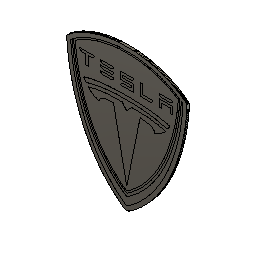
Tesla Shield Multipart (Autodesk Fusion 360 design; units mm, degrees)
Autodesk Fusion 360 part; units mm, degrees
(part 1 of 3)
sketch "Tesla Shield" plane through (0, 0, 0) normal (0, 0, 1) x (1, 0, 0)
  line L0 (187.3472, 241.9811) -> (187.8279, 240.6292)
  line L1 (217.7382, 211.8612) -> (216.8697, 213.1105)
  line L2 (210.0287, 224.007) -> (209.4066, 225.0419)
  line L3 (226.1937, 201.0406) -> (225.1992, 202.2018)
  line L4 (206.605, 201.6349) -> (207.38, 200.4172)
  line L5 (185.9594, 246.0449) -> (186.4129, 244.6891)
  line L6 (196.7783, 219.3402) -> (197.4176, 218.0403)
  line L7 (208.9597, 198.0038) -> (209.7645, 196.8085)
  line L8 (211.4038, 194.4412) -> (212.2385, 193.2697)
  line L9 (225.9747, 176.798) -> (226.9727, 175.7815)
  line L10 (228.9998, 173.7824) -> (230.029, 172.8002)
  line L11 (201.773, 240.4243) -> (201.2849, 241.5783)
  line L12 (192.5686, 228.5557) -> (193.1417, 227.228)
  line L13 (185.0795, 248.7587) -> (185.5149, 247.4014)
  line L14 (194.3162, 224.5831) -> (194.9175, 223.2662)
  line L15 (200.8071, 242.7368) -> (199.8754, 245.0637)
  line L16 (209.4066, 225.0419) -> (208.7947, 226.0826)
  line L17 (184.653, 250.1165) -> (185.0795, 248.7587)
  line L18 (224.218, 203.374) -> (223.2505, 204.5568)
  line L19 (193.7243, 225.9038) -> (194.3162, 224.5831)
  line L20 (197.4176, 218.0403) -> (198.0664, 216.745)
  line L21 (220.2044, 183.1227) -> (221.1404, 182.0426)
  line L22 (189.3251, 236.5837) -> (189.8425, 235.2392)
  line L23 (221.1404, 182.0426) -> (222.0866, 180.9727)
  line L24 (218.3631, 185.3125) -> (219.2786, 184.2127)
  line L25 (213.0832, 192.1065) -> (213.9379, 190.9519)
  line L26 (208.7947, 226.0826) -> (208.4968, 226.6074)
  line L27 (185.5149, 247.4014) -> (185.9594, 246.0449)
  line L28 (192.0048, 229.8867) -> (192.5686, 228.5557)
  line L29 (200.7575, 211.6148) -> (201.4543, 210.3458)
  line L30 (201.4543, 210.3458) -> (202.1609, 209.0826)
  line L31 (212.4736, 219.9224) -> (211.5554, 221.4433)
  line L32 (202.7875, 238.1331) -> (202.2733, 239.2756)
  line L33 (246.8929, 159.2455) -> (247.0305, 159.1815)
  line L34 (191.4503, 231.2207) -> (192.0048, 229.8867)
  line L35 (202.8772, 207.8253) -> (203.6032, 206.5742)
  line L36 (236.2567, 167.2973) -> (237.1439, 166.5675)
  line L37 (188.3178, 239.2788) -> (188.8169, 237.9302)
  line L38 (213.4053, 218.4097) -> (212.4736, 219.9224)
  line L39 (227.981, 174.7763) -> (228.9998, 173.7824)
  line L40 (205.0845, 204.0912) -> (205.8398, 202.8596)
  line L41 (195.5283, 221.9533) -> (196.1486, 220.6446)
  line L42 (220.4307, 208.1662) -> (219.5188, 209.3888)
  line L43 (186.4129, 244.6891) -> (186.8755, 243.3345)
  line L44 (189.8425, 235.2392) -> (190.3692, 233.8971)
  line L45 (188.8169, 237.9302) -> (189.3251, 236.5837)
  line L46 (202.2733, 239.2756) -> (201.773, 240.4243)
  line L47 (186.8755, 243.3345) -> (187.3472, 241.9811)
  line L48 (194.9175, 223.2662) -> (195.5283, 221.9533)
  line L49 (193.1417, 227.228) -> (193.7243, 225.9038)
  line L50 (227.2015, 199.8907) -> (226.1937, 201.0406)
  line L51 (198.7247, 215.4547) -> (199.3927, 214.1694)
  line L52 (190.9051, 232.5575) -> (191.4503, 231.2207)
  line L53 (216.8697, 213.1105) -> (216.0159, 214.3681)
  line L54 (214.3531, 216.9072) -> (213.4053, 218.4097)
  line L55 (208.4968, 226.6074) -> (208.2063, 227.1364)
  line L56 (199.8754, 245.0637) -> (198.9639, 247.3984)
  line L57 (211.5554, 221.4433) -> (210.648, 222.9706)
  line L58 (223.2505, 204.5568) -> (222.2966, 205.7499)
  line L59 (201.2849, 241.5783) -> (200.8071, 242.7368)
  line L60 (200.0703, 212.8894) -> (200.7575, 211.6148)
  line L61 (245.9016, 159.8961) -> (246.3605, 159.5744)
  line L62 (225.1992, 202.2018) -> (224.218, 203.374)
  line L63 (216.0159, 214.3681) -> (215.177, 215.6338)
  line L64 (213.9379, 190.9519) -> (214.8027, 189.8059)
  line L65 (245.3558, 160.2891) -> (245.9016, 159.8961)
  line L66 (246.7357, 159.3331) -> (246.8929, 159.2455)
  line L67 (234.5005, 168.7781) -> (235.3754, 168.0341)
  line L68 (216.5626, 187.5407) -> (217.4578, 186.4219)
  line L69 (207.38, 200.4172) -> (208.1649, 199.2068)
  line L70 (224.01, 178.864) -> (224.9872, 177.8256)
  line L71 (235.3754, 168.0341) -> (236.2567, 167.2973)
  line L72 (240.7476, 163.7156) -> (241.6609, 163.0186)
  line L73 (233.6321, 169.5295) -> (234.5005, 168.7781)
  line L74 (203.6032, 206.5742) -> (204.3389, 205.3294)
  line L75 (239.8389, 164.4189) -> (240.7476, 163.7156)
  line L76 (241.6609, 163.0186) -> (243.5005, 161.6424)
  line L77 (205.8398, 202.8596) -> (206.605, 201.6349)
  line L78 (226.9727, 175.7815) -> (227.981, 174.7763)
  line L79 (243.5005, 161.6424) -> (245.3558, 160.2891)
  line L80 (209.7645, 196.8085) -> (210.5791, 195.6209)
  line L81 (237.1439, 166.5675) -> (238.0368, 165.8447)
  line L82 (238.9353, 165.1285) -> (239.8389, 164.4189)
  line L83 (210.5791, 195.6209) -> (211.4038, 194.4412)
  line L84 (215.6776, 188.6688) -> (216.5626, 187.5407)
  line L85 (231.9159, 171.0551) -> (232.7705, 170.2885)
  line L86 (223.0431, 179.9131) -> (224.01, 178.864)
  line L87 (217.4578, 186.4219) -> (218.3631, 185.3125)
  line L88 (222.0866, 180.9727) -> (223.0431, 179.9131)
  line L89 (231.0687, 171.8297) -> (231.9159, 171.0551)
  line L90 (246.3605, 159.5744) -> (246.7357, 159.3331)
  line L91 (219.2786, 184.2127) -> (220.2044, 183.1227)
  line L92 (208.1649, 199.2068) -> (208.9597, 198.0038)
  line L93 (238.0368, 165.8447) -> (238.9353, 165.1285)
  line L94 (230.029, 172.8002) -> (231.0687, 171.8297)
  line L95 (212.2385, 193.2697) -> (213.0832, 192.1065)
  line L96 (214.8027, 189.8059) -> (215.6776, 188.6688)
  line L97 (232.7705, 170.2885) -> (233.6321, 169.5295)
  line L98 (224.9872, 177.8256) -> (225.9747, 176.798)
  line L99 (204.3389, 205.3294) -> (205.0845, 204.0912)
  line L100 (297.8145, 269.3775) -> (297.8286, 269.41)
  line L101 (206.9505, 271.3462) -> (206.1166, 271.1382)
  line L102 (220.5752, 273.5951) -> (218.9108, 273.3996)
  line L103 (244.7346, 273.0159) -> (244.2152, 273.6532)
  line L104 (200.9819, 269.6639) -> (200.9198, 269.6275)
  line L105 (293.8572, 265.8465) -> (294.3752, 266.2321)
  line L106 (263.8971, 274.4151) -> (262.0411, 274.448)
  line L107 (255.4396, 274.4952) -> (255.1595, 274.4828)
  line L108 (227.5104, 274.2394) -> (226.7191, 274.1886)
  line L109 (260.1865, 274.4663) -> (258.0237, 274.484)
  line L110 (201.2563, 268.8271) -> (201.3792, 268.686)
  line L111 (202.4895, 270.1206) -> (201.6512, 269.8782)
  line L112 (248.9154, 267.9355) -> (248.592, 268.3323)
  line L113 (226.7191, 274.1886) -> (225.7816, 274.1169)
  line L114 (243.5571, 274.4237) -> (243.4699, 274.5089)
  line L115 (249.1841, 267.626) -> (249.1226, 267.6892)
  line L116 (282.4148, 273.0309) -> (280.5744, 273.2723)
  line L117 (293.3298, 265.4726) -> (293.8572, 265.8465)
  line L118 (212.9583, 261.2685) -> (214.347, 260.9395)
  line L119 (265.7539, 274.3663) -> (263.8971, 274.4151)
  line L120 (219.1338, 266.4225) -> (219.4722, 266.55)
  line L121 (288.8178, 271.9664) -> (287.9073, 272.1405)
  line L122 (203.8665, 266.4028) -> (204.2509, 266.108)
  line L123 (212.8487, 272.5505) -> (212.0009, 272.4036)
  line L124 (297.8286, 269.41) -> (295.7733, 270.2687)
  line L125 (216.9125, 265.358) -> (217.2645, 265.5571)
  line L126 (202.0493, 267.9939) -> (202.3973, 267.6598)
  line L127 (208.7098, 263.3768) -> (209.7655, 262.8217)
  line L128 (269.4679, 274.2167) -> (267.611, 274.3005)
  line L129 (216.6366, 265.1892) -> (216.9125, 265.358)
  line L130 (249.1226, 267.6892) -> (248.9154, 267.9355)
  line L131 (200.9245, 269.36) -> (200.978, 269.2386)
  line L132 (295.8664, 267.4615) -> (296.3401, 267.8965)
  line L133 (267.611, 274.3005) -> (265.7539, 274.3663)
  line L134 (214.347, 260.9395) -> (214.6904, 262.7698)
  line L135 (216.2433, 264.9136) -> (216.4345, 265.0556)
  line L136 (289.7268, 271.7846) -> (288.8178, 271.9664)
  line L137 (203.1174, 267.0156) -> (203.4885, 266.7053)
  line L138 (258.0237, 274.484) -> (256.4399, 274.4982)
  line L139 (286.9953, 272.307) -> (286.0818, 272.4661)
  line L140 (294.3752, 266.2321) -> (294.8833, 266.6296)
  line L141 (297.5669, 269.108) -> (297.7654, 269.3164)
  line L142 (203.6318, 270.4539) -> (202.4895, 270.1206)
  line L143 (217.2645, 265.5571) -> (217.6947, 265.7815)
  line L144 (243.8236, 274.1236) -> (243.5571, 274.4237)
  line L145 (249.2182, 267.6047) -> (249.1841, 267.626)
  line L146 (248.1479, 268.8686) -> (247.0886, 270.1383)
  line L147 (295.3806, 267.0393) -> (295.8664, 267.4615)
  line L148 (200.8951, 269.4677) -> (200.9245, 269.36)
  line L149 (218.7986, 266.2867) -> (219.1338, 266.4225)
  line L150 (204.457, 270.6923) -> (203.6318, 270.4539)
  line L151 (255.0748, 274.4732) -> (255.0271, 274.461)
  line L152 (280.5744, 273.2723) -> (278.7301, 273.4878)
  line L153 (248.592, 268.3323) -> (248.1479, 268.8686)
  line L154 (209.4669, 271.9142) -> (208.6259, 271.734)
  line L155 (273.1788, 273.9905) -> (271.324, 274.1137)
  line L156 (201.7098, 268.3359) -> (202.0493, 267.9939)
  line L157 (287.9073, 272.1405) -> (286.9953, 272.307)
  line L158 (202.7535, 267.3338) -> (203.1174, 267.0156)
  line L159 (286.0818, 272.4661) -> (284.2508, 272.7625)
  line L160 (255.0271, 274.461) -> (249.2182, 267.6047)
  line L161 (262.0411, 274.448) -> (260.1865, 274.4663)
  line L162 (207.5087, 264.0243) -> (208.7098, 263.3768)
  line L163 (278.7301, 273.4878) -> (276.8823, 273.6786)
  line L164 (252.6831, 166.1124) -> (253.7398, 166.8931)
  line L165 (203.4885, 266.7053) -> (203.8665, 266.4028)
  line L166 (226.8539, 268.0985) -> (232.4298, 268.1876)
  line L167 (211.4348, 261.9774) -> (212.5034, 261.4676)
  line L168 (219.8135, 266.6699) -> (220.1574, 266.7825)
  line L169 (200.9023, 269.5956) -> (200.8926, 269.558)
  line L170 (218.2053, 266.0263) -> (218.7986, 266.2867)
  line L171 (212.5034, 261.4676) -> (212.9583, 261.2685)
  line L172 (232.5255, 268.105) -> (232.5909, 267.9917)
  line L173 (200.8926, 269.558) -> (200.8951, 269.4677)
  line L174 (250.0262, 164.2337) -> (250.3806, 164.4663)
  line L175 (204.2509, 266.108) -> (204.6414, 265.821)
  line L176 (273.2336, 184.725) -> (274.0907, 185.682)
  line L177 (232.4822, 268.1528) -> (232.5255, 268.105)
  line L178 (200.9198, 269.6275) -> (200.9023, 269.5956)
  line L179 (201.3792, 268.686) -> (201.7098, 268.3359)
  line L180 (206.1166, 271.1382) -> (205.2853, 270.9203)
  line L181 (201.6512, 269.8782) -> (201.1251, 269.717)
  line L182 (217.1017, 273.1756) -> (215.3984, 272.9463)
  line L183 (207.0877, 264.2585) -> (207.5087, 264.0243)
  line L184 (255.8253, 168.4921) -> (256.8568, 169.3066)
  line L185 (224.4041, 267.7293) -> (225.0148, 267.8346)
  line L186 (225.0148, 267.8346) -> (225.6259, 267.9391)
  line L187 (250.3806, 164.4663) -> (250.7648, 164.7364)
  line L188 (251.6155, 165.3469) -> (252.6831, 166.1124)
  line L189 (253.7398, 166.8931) -> (254.7867, 167.687)
  line L190 (215.3984, 272.9463) -> (213.6976, 272.6897)
  line L191 (200.978, 269.2386) -> (201.053, 269.1069)
  line L192 (205.0375, 265.5417) -> (205.4388, 265.27)
  line L193 (201.1251, 269.717) -> (200.9819, 269.6639)
  line L194 (202.3973, 267.6598) -> (202.7535, 267.3338)
  line L195 (210.3099, 272.0857) -> (209.4669, 271.9142)
  line L196 (205.4388, 265.27) -> (205.8449, 265.0059)
  line L197 (232.6262, 267.8904) -> (232.673, 267.7116)
  line L198 (249.1594, 163.8662) -> (249.2821, 163.8853)
  line L199 (249.5544, 163.9782) -> (249.7034, 164.0492)
  line L200 (221.5548, 267.1691) -> (222.2632, 267.3304)
  line L201 (219.4722, 266.55) -> (219.8135, 266.6699)
  line L202 (254.7867, 167.687) -> (255.8253, 168.4921)
  line L203 (225.6259, 267.9391) -> (226.2385, 268.0311)
  line L204 (250.7648, 164.7364) -> (251.6155, 165.3469)
  line L205 (218.9108, 273.3996) -> (217.1017, 273.1756)
  line L206 (214.6904, 262.7698) -> (216.2433, 264.9136)
  line L207 (212.0009, 272.4036) -> (211.1546, 272.2488)
  line L208 (213.6976, 272.6897) -> (212.8487, 272.5505)
  line L209 (206.2553, 264.7493) -> (206.6697, 264.5002)
  line L210 (210.6744, 262.3563) -> (211.4348, 261.9774)
  line L211 (247.7838, 192.4016) -> (248.8733, 187.0975)
  line L212 (216.4345, 265.0556) -> (216.6366, 265.1892)
  line L213 (272.4031, 183.8146) -> (273.2336, 184.725)
  line L214 (205.8449, 265.0059) -> (206.2553, 264.7493)
  line L215 (206.6697, 264.5002) -> (207.0877, 264.2585)
  line L216 (249.2821, 163.8853) -> (249.4139, 163.9231)
  line L217 (209.7655, 262.8217) -> (210.6744, 262.3563)
  line L218 (217.6947, 265.7815) -> (218.2053, 266.0263)
  line L219 (211.1546, 272.2488) -> (210.3099, 272.0857)
  line L220 (208.6259, 271.734) -> (207.787, 271.5448)
  line L221 (207.787, 271.5448) -> (206.9505, 271.3462)
  line L222 (201.1467, 268.9685) -> (201.2563, 268.8271)
  line L223 (204.6414, 265.821) -> (205.0375, 265.5417)
  line L224 (233.2192, 265.0188) -> (233.8646, 261.69)
  line L225 (232.673, 267.7116) -> (232.803, 267.1221)
  line L226 (201.053, 269.1069) -> (201.1467, 268.9685)
  line L227 (205.2853, 270.9203) -> (204.457, 270.6923)
  line L228 (264.0551, 175.3271) -> (264.7286, 175.9763)
  line L229 (300.0785, 226.3396) -> (300.6089, 227.5112)
  line L230 (222.2632, 267.3304) -> (222.9755, 267.4752)
  line L231 (249.0458, 163.8669) -> (249.1594, 163.8662)
  line L232 (222.9755, 267.4752) -> (223.6898, 267.6069)
  line L233 (261.4587, 173.0304) -> (262.2197, 173.6613)
  line L234 (226.2385, 268.0311) -> (226.5458, 268.0686)
  line L235 (267.2612, 178.4867) -> (269.3757, 180.6291)
  line L236 (270.0856, 181.3582) -> (270.8278, 182.1318)
  line L237 (278.7265, 191.1855) -> (279.714, 192.4337)
  line L238 (291.3793, 209.609) -> (292.4763, 211.4976)
  line L239 (316.644, 280.0686) -> (316.9675, 281.8919)
  line L240 (248.9417, 163.8888) -> (249.0458, 163.8669)
  line L241 (234.2811, 259.5685) -> (234.7645, 257.1438)
  line L242 (296.3072, 218.5588) -> (296.851, 219.6258)
  line L243 (281.738, 195.0818) -> (282.7718, 196.4828)
  line L244 (316.3068, 278.247) -> (316.644, 280.0686)
  line L245 (279.714, 192.4337) -> (280.7183, 193.7323)
  line L246 (299.5457, 225.1831) -> (300.0785, 226.3396)
  line L247 (275.8791, 187.738) -> (276.8077, 188.8382)
  line L248 (284.8759, 199.4415) -> (285.9434, 201.0002)
  line L249 (304.6788, 237.2471) -> (305.3427, 238.9769)
  line L250 (313.5607, 265.5564) -> (313.9947, 267.3614)
  line L251 (283.8182, 197.9359) -> (284.8759, 199.4415)
  line L252 (243.375, 214.2341) -> (246.5055, 198.6926)
  line L253 (220.1574, 266.7825) -> (220.8522, 266.9876)
  line L254 (226.5458, 268.0686) -> (226.8539, 268.0985)
  line L255 (249.7034, 164.0492) -> (250.0262, 164.2337)
  line L256 (256.8568, 169.3066) -> (257.8825, 170.1284)
  line L257 (264.7286, 175.9763) -> (265.4875, 176.7193)
  line L258 (262.9646, 174.3106) -> (263.4671, 174.7719)
  line L259 (234.7645, 257.1438) -> (239.4665, 233.7189)
  line L260 (239.4665, 233.7189) -> (243.375, 214.2341)
  line L261 (249.4139, 163.9231) -> (249.5544, 163.9782)
  line L262 (265.4875, 176.7193) -> (267.2612, 178.4867)
  line L263 (297.3935, 220.7075) -> (297.9343, 221.804)
  line L264 (271.6007, 182.9504) -> (272.4031, 183.8146)
  line L265 (297.9343, 221.804) -> (298.4734, 222.9154)
  line L266 (310.6609, 254.8005) -> (311.1797, 256.5833)
  line L267 (295.2162, 216.4689) -> (295.7622, 217.5066)
  line L268 (287.0193, 202.6126) -> (288.1022, 204.2791)
  line L269 (316.9675, 281.8919) -> (317.2775, 283.7165)
  line L270 (270.8278, 182.1318) -> (271.6007, 182.9504)
  line L271 (314.4147, 269.1693) -> (314.8208, 270.9801)
  line L272 (220.8522, 266.9876) -> (221.5548, 267.1691)
  line L273 (232.4298, 268.1876) -> (232.4822, 268.1528)
  line L274 (223.6898, 267.6069) -> (224.4041, 267.7293)
  line L275 (257.8825, 170.1284) -> (259.9219, 171.7863)
  line L276 (259.9219, 171.7863) -> (260.69, 172.4086)
  line L277 (262.5946, 173.983) -> (262.9646, 174.3106)
  line L278 (314.8208, 270.9801) -> (315.213, 272.7934)
  line L279 (232.803, 267.1221) -> (233.2192, 265.0188)
  line L280 (317.2775, 283.7165) -> (317.5739, 285.5423)
  line L281 (232.5909, 267.9917) -> (232.6262, 267.8904)
  line L282 (262.2197, 173.6613) -> (262.5946, 173.983)
  line L283 (263.4671, 174.7719) -> (264.0551, 175.3271)
  line L284 (246.5055, 198.6926) -> (247.7838, 192.4016)
  line L285 (260.69, 172.4086) -> (261.4587, 173.0304)
  line L286 (233.8646, 261.69) -> (234.2811, 259.5685)
  line L287 (269.3757, 180.6291) -> (270.0856, 181.3582)
  line L288 (292.4763, 211.4976) -> (293.5735, 213.443)
  line L289 (312.6507, 261.9562) -> (313.1127, 263.7546)
  line L290 (306.6263, 242.455) -> (307.2462, 244.2028)
  line L291 (311.057, 269.1781) -> (310.5368, 267.2186)
  line L292 (301.8749, 230.3938) -> (302.5982, 232.0968)
  line L293 (309.0185, 249.4792) -> (309.5804, 251.2482)
  line L294 (289.1908, 206.0003) -> (290.2836, 207.7768)
  line L295 (315.5914, 274.6092) -> (315.956, 276.4271)
  line L296 (318.2833, 311.6756) -> (318.1327, 311.7716)
  line L297 (318.9513, 295.7252) -> (319.1769, 297.7683)
  line L298 (318.0583, 311.8056) -> (317.9875, 311.8223)
  line L299 (305.9918, 240.7129) -> (306.6263, 242.455)
  line L300 (317.0429, 301.2385) -> (316.7655, 298.9748)
  line L301 (318.7104, 293.6839) -> (318.9513, 295.7252)
  line L302 (313.9947, 267.3614) -> (314.4147, 269.1693)
  line L303 (305.3427, 238.9769) -> (305.9918, 240.7129)
  line L304 (317.8858, 287.5735) -> (318.1786, 289.6077)
  line L305 (290.2836, 207.7768) -> (291.3793, 209.609)
  line L306 (317.5739, 285.5423) -> (317.8858, 287.5735)
  line L307 (317.9875, 311.8223) -> (317.9226, 311.8158)
  line L308 (317.8512, 311.717) -> (317.8513, 311.5749)
  line L309 (317.9226, 311.8158) -> (317.8929, 311.802)
  line L310 (303.3066, 233.8068) -> (304.0001, 235.5236)
  line L311 (312.1745, 260.1614) -> (312.6507, 261.9562)
  line L312 (317.8562, 311.7585) -> (317.8512, 311.717)
  line L313 (311.1797, 256.5833) -> (311.6842, 258.3704)
  line L314 (274.973, 186.6861) -> (275.8791, 187.738)
  line L315 (319.8105, 304.1054) -> (319.9099, 305.2299)
  line L316 (308.4423, 247.7151) -> (309.0185, 249.4792)
  line L317 (307.2462, 244.2028) -> (307.8515, 245.9563)
  line L318 (276.8077, 188.8382) -> (277.7573, 189.9872)
  line L319 (315.956, 276.4271) -> (316.3068, 278.247)
  line L320 (293.5735, 213.443) -> (294.6692, 215.4458)
  line L321 (319.5848, 310.7886) -> (319.3691, 310.9524)
  line L322 (317.8656, 309.1223) -> (317.7995, 308.2954)
  line L323 (274.0907, 185.682) -> (274.973, 186.6861)
  line L324 (317.6106, 306.3265) -> (317.4624, 304.9147)
  line L325 (313.1127, 263.7546) -> (313.5607, 265.5564)
  line L326 (318.4531, 291.6446) -> (318.7104, 293.6839)
  line L327 (301.1367, 228.698) -> (301.8749, 230.3938)
  line L328 (280.7183, 193.7323) -> (281.738, 195.0818)
  line L329 (299.0106, 224.0417) -> (299.5457, 225.1831)
  line L330 (295.7622, 217.5066) -> (296.3072, 218.5588)
  line L331 (315.213, 272.7934) -> (315.5914, 274.6092)
  line L332 (309.4434, 263.3145) -> (308.8702, 261.3705)
  line L333 (317.8932, 310.238) -> (317.8878, 309.7166)
  line L334 (308.2793, 259.4321) -> (307.6706, 257.4998)
  line L335 (319.9796, 306.3562) -> (319.9823, 310.4304)
  line L336 (317.8929, 311.802) -> (317.8656, 311.7802)
  line L337 (310.1278, 253.0221) -> (310.6609, 254.8005)
  line L338 (300.6089, 227.5112) -> (301.1367, 228.698)
  line L339 (311.6842, 258.3704) -> (312.1745, 260.1614)
  line L340 (317.8745, 311.0582) -> (317.887, 310.6855)
  line L341 (285.9434, 201.0002) -> (287.0193, 202.6126)
  line L342 (282.7718, 196.4828) -> (283.8182, 197.9359)
  line L343 (309.5804, 251.2482) -> (310.1278, 253.0221)
  line L344 (298.4734, 222.9154) -> (299.0106, 224.0417)
  line L345 (302.5982, 232.0968) -> (303.3066, 233.8068)
  line L346 (294.6692, 215.4458) -> (295.2162, 216.4689)
  line L347 (288.1022, 204.2791) -> (289.1908, 206.0003)
  line L348 (307.8515, 245.9563) -> (308.4423, 247.7151)
  line L349 (277.7573, 189.9872) -> (278.7265, 191.1855)
  line L350 (304.0001, 235.5236) -> (304.6788, 237.2471)
  line L351 (296.851, 219.6258) -> (297.3935, 220.7075)
  line L352 (319.5859, 301.8583) -> (319.6973, 302.9819)
  line L353 (319.7526, 310.6519) -> (319.5848, 310.7886)
  line L354 (253.4077, 176.8014) -> (252.5487, 176.1361)
  line L355 (254.4425, 177.5977) -> (253.4077, 176.8014)
  line L356 (276.3342, 198.274) -> (275.6602, 197.4383)
  line L357 (278.4805, 200.9452) -> (277.3614, 199.5409)
  line L358 (312.5122, 275.0833) -> (312.0447, 273.1107)
  line L359 (319.3691, 310.9524) -> (319.1042, 311.1409)
  line L360 (314.2075, 283.0089) -> (313.8098, 281.0227)
  line L361 (319.1042, 311.1409) -> (318.7888, 311.3516)
  line L362 (316.5061, 296.9742) -> (316.2295, 294.9744)
  line L363 (319.9099, 305.2299) -> (319.9495, 305.7927)
  line L364 (312.9622, 277.0596) -> (312.5122, 275.0833)
  line L365 (319.9823, 310.4304) -> (319.9501, 310.4703)
  line L366 (318.7888, 311.3516) -> (318.4215, 311.5819)
  line L367 (319.9501, 310.4703) -> (319.8739, 310.545)
  line L368 (319.9495, 305.7927) -> (319.9796, 306.3562)
  line L369 (314.5878, 284.9979) -> (314.2075, 283.0089)
  line L370 (293.9809, 224.7423) -> (293.153, 223.207)
  line L371 (277.3614, 199.5409) -> (276.3342, 198.274)
  line L372 (317.7995, 308.2954) -> (317.6106, 306.3265)
  line L373 (248.8628, 174.2348) -> (248.4253, 174.5107)
  line L374 (285.9584, 211.2601) -> (285.2039, 210.1338)
  line L375 (319.3881, 299.8128) -> (319.5859, 301.8583)
  line L376 (251.3229, 175.2514) -> (249.0538, 174.1399)
  line L377 (260.9178, 182.6508) -> (259.8842, 181.8192)
  line L378 (316.2295, 294.9744) -> (315.9357, 292.9758)
  line L379 (257.4241, 179.8877) -> (255.9983, 178.7876)
  line L380 (319.8739, 310.545) -> (319.7526, 310.6519)
  line L381 (317.8878, 309.7166) -> (317.8656, 309.1223)
  line L382 (306.3999, 253.6539) -> (305.7378, 251.741)
  line L383 (319.1769, 297.7683) -> (319.3881, 299.8128)
  line L384 (318.1786, 289.6077) -> (318.4531, 291.6446)
  line L385 (317.2742, 303.2186) -> (317.0429, 301.2385)
  line L386 (317.887, 310.6855) -> (317.8932, 310.238)
  line L387 (317.8656, 311.7802) -> (317.8562, 311.7585)
  line L388 (317.4624, 304.9147) -> (317.2742, 303.2186)
  line L389 (313.8098, 281.0227) -> (313.3947, 279.0396)
  line L390 (302.1587, 242.2871) -> (301.389, 240.4204)
  line L391 (315.2963, 288.9829) -> (314.9507, 286.9893)
  line L392 (259.8842, 181.8192) -> (258.7195, 180.8983)
  line L393 (305.7378, 251.741) -> (305.0579, 249.8351)
  line L394 (311.5596, 271.1423) -> (311.057, 269.1781)
  line L395 (315.6246, 290.9785) -> (315.2963, 288.9829)
  line L396 (313.3947, 279.0396) -> (312.9622, 277.0596)
  line L397 (315.9357, 292.9758) -> (315.6246, 290.9785)
  line L398 (319.6973, 302.9819) -> (319.8105, 304.1054)
  line L399 (317.8513, 311.5749) -> (317.8745, 311.0582)
  line L400 (312.0447, 273.1107) -> (311.5596, 271.1423)
  line L401 (309.9989, 265.264) -> (309.4434, 263.3145)
  line L402 (316.7655, 298.9748) -> (316.5061, 296.9742)
  line L403 (314.9507, 286.9893) -> (314.5878, 284.9979)
  line L404 (318.1327, 311.7716) -> (318.0583, 311.8056)
  line L405 (248.4253, 174.5107) -> (247.7448, 174.9666)
  line L406 (310.5368, 267.2186) -> (309.9989, 265.264)
  line L407 (308.8702, 261.3705) -> (308.2793, 259.4321)
  line L408 (274.9876, 196.6014) -> (274.3041, 195.7739)
  line L409 (300.6011, 238.5623) -> (299.7953, 236.7131)
  line L410 (292.3283, 221.7142) -> (291.5079, 220.2636)
  line L411 (302.9105, 244.1622) -> (302.1587, 242.2871)
  line L412 (286.7242, 212.4257) -> (285.9584, 211.2601)
  line L413 (274.3041, 195.7739) -> (273.9544, 195.3671)
  line L414 (263.2292, 184.6098) -> (262.5907, 184.046)
  line L415 (284.4617, 209.0463) -> (283.7327, 207.9972)
  line L416 (318.4215, 311.5819) -> (318.2833, 311.6756)
  line L417 (262.5907, 184.046) -> (261.8201, 183.393)
  line L418 (218.5367, 202.9667) -> (217.8938, 203.8125)
  line L419 (203.744, 226.3267) -> (202.7719, 228.2187)
  line L420 (196.63, 241.7002) -> (196.0544, 243.1275)
  line L421 (225.2918, 194.8006) -> (224.5897, 195.592)
  line L422 (246.825, 175.6017) -> (245.9952, 176.1865)
  line L423 (252.5487, 176.1361) -> (251.8567, 175.6151)
  line L424 (275.6602, 197.4383) -> (274.9876, 196.6014)
  line L425 (228.1596, 191.6954) -> (227.4338, 192.4625)
  line L426 (285.2039, 210.1338) -> (284.4617, 209.0463)
  line L427 (210.0741, 215.2243) -> (208.9599, 217.0414)
  line L428 (194.9347, 245.9959) -> (194.3907, 247.4369)
  line L429 (283.7327, 207.9972) -> (283.0176, 206.9863)
  line L430 (221.8403, 198.8151) -> (221.1677, 199.6348)
  line L431 (195.4893, 244.5594) -> (194.9347, 245.9959)
  line L432 (305.0579, 249.8351) -> (304.36, 247.9365)
  line L433 (197.4364, 239.7539) -> (196.63, 241.7002)
  line L434 (255.9983, 178.7876) -> (254.4425, 177.5977)
  line L435 (223.8934, 196.3892) -> (223.2031, 197.1922)
  line L436 (251.8567, 175.6151) -> (251.5706, 175.4127)
  line L437 (280.9657, 204.1784) -> (279.6844, 202.4901)
  line L438 (281.6333, 205.0772) -> (280.9657, 204.1784)
  line L439 (296.476, 229.6075) -> (295.6433, 227.9422)
  line L440 (294.8114, 226.3206) -> (293.9809, 224.7423)
  line L441 (307.0442, 255.5736) -> (306.3999, 253.6539)
  line L442 (295.6433, 227.9422) -> (294.8114, 226.3206)
  line L443 (198.2664, 237.8132) -> (197.4364, 239.7539)
  line L444 (196.0544, 243.1275) -> (195.4893, 244.5594)
  line L445 (298.1396, 233.0707) -> (297.3084, 231.3168)
  line L446 (297.3084, 231.3168) -> (296.476, 229.6075)
  line L447 (303.6442, 246.0455) -> (302.9105, 244.1622)
  line L448 (239.547, 181.1306) -> (238.7646, 181.7791)
  line L449 (273.5973, 194.9667) -> (263.2292, 184.6098)
  line L450 (288.2864, 214.876) -> (287.5005, 213.6309)
  line L451 (240.3346, 180.4884) -> (239.547, 181.1306)
  line L452 (242.7289, 178.6019) -> (241.9255, 179.2239)
  line L453 (299.7953, 236.7131) -> (298.9689, 234.8693)
  line L454 (247.7448, 174.9666) -> (246.825, 175.6017)
  line L455 (289.081, 216.1615) -> (288.2864, 214.876)
  line L456 (279.6844, 202.4901) -> (278.4805, 200.9452)
  line L457 (290.6926, 218.8549) -> (289.8834, 217.4877)
  line L458 (283.0176, 206.9863) -> (282.3176, 206.0131)
  line L459 (261.8201, 183.393) -> (260.9178, 182.6508)
  line L460 (245.1707, 176.7791) -> (244.3514, 177.3793)
  line L461 (249.0538, 174.1399) -> (248.9893, 174.1647)
  line L462 (298.9689, 234.8693) -> (298.1396, 233.0707)
  line L463 (287.5005, 213.6309) -> (286.7242, 212.4257)
  line L464 (221.1677, 199.6348) -> (220.5011, 200.4599)
  line L465 (216.6256, 205.5188) -> (216.0004, 206.3792)
  line L466 (243.5375, 177.987) -> (242.7289, 178.6019)
  line L467 (233.4062, 186.5077) -> (232.6389, 187.2287)
  line L468 (273.9544, 195.3671) -> (273.5973, 194.9667)
  line L469 (307.6706, 257.4998) -> (307.0442, 255.5736)
  line L470 (251.5706, 175.4127) -> (251.3229, 175.2514)
  line L471 (304.36, 247.9365) -> (303.6442, 246.0455)
  line L472 (289.8834, 217.4877) -> (289.081, 216.1615)
  line L473 (282.3176, 206.0131) -> (281.6333, 205.0772)
  line L474 (248.9893, 174.1647) -> (248.8628, 174.2348)
  line L475 (301.389, 240.4204) -> (300.6011, 238.5623)
  line L476 (291.5079, 220.2636) -> (290.6926, 218.8549)
  line L477 (258.7195, 180.8983) -> (257.4241, 179.8877)
  line L478 (293.153, 223.207) -> (292.3283, 221.7142)
  line L479 (206.8025, 220.7177) -> (205.7593, 222.5755)
  line L480 (205.7593, 222.5755) -> (204.7398, 224.4454)
  line L481 (217.2567, 204.6632) -> (216.6256, 205.5188)
  line L482 (180.9601, 306.9902) -> (180.7887, 308.9699)
  line L483 (179.5198, 311.1773) -> (179.2171, 310.994)
  line L484 (190.4109, 259.1095) -> (189.9595, 260.5849)
  line L485 (245.9952, 176.1865) -> (245.1707, 176.7791)
  line L486 (223.2031, 197.1922) -> (222.5187, 198.0008)
  line L487 (229.629, 190.1803) -> (228.8914, 190.9347)
  line L488 (211.212, 213.4223) -> (210.0741, 215.2243)
  line L489 (234.1793, 185.7936) -> (233.4062, 186.5077)
  line L490 (225.9999, 194.0152) -> (225.2918, 194.8006)
  line L491 (237.9874, 182.4338) -> (237.2155, 183.0945)
  line L492 (217.8938, 203.8125) -> (217.2567, 204.6632)
  line L493 (220.5011, 200.4599) -> (219.8404, 201.2903)
  line L494 (235.6871, 184.4331) -> (234.1793, 185.7936)
  line L495 (219.8404, 201.2903) -> (219.1856, 202.126)
  line L496 (207.8694, 218.8728) -> (206.8025, 220.7177)
  line L497 (208.9599, 217.0414) -> (207.8694, 218.8728)
  line L498 (228.8914, 190.9347) -> (228.1596, 191.6954)
  line L499 (200.8986, 232.0318) -> (199.9976, 233.9514)
  line L500 (236.4487, 183.761) -> (235.6871, 184.4331)
  line L501 (216.0004, 206.3792) -> (214.7678, 208.1138)
  line L502 (231.8775, 187.9565) -> (231.1221, 188.6911)
  line L503 (241.1274, 179.8528) -> (240.3346, 180.4884)
  line L504 (232.6389, 187.2287) -> (231.8775, 187.9565)
  line L505 (180.5485, 311.4822) -> (180.5241, 311.5848)
  line L506 (179.1889, 302.9124) -> (179.4131, 300.5317)
  line L507 (191.3441, 256.1689) -> (190.8724, 257.6375)
  line L508 (224.5897, 195.592) -> (223.8934, 196.3892)
  line L509 (238.7646, 181.7791) -> (237.9874, 182.4338)
  line L510 (183.533, 287.5775) -> (183.2681, 289.0936)
  line L511 (199.1202, 235.8788) -> (198.2664, 237.8132)
  line L512 (231.1221, 188.6911) -> (230.3726, 189.4324)
  line L513 (204.7398, 224.4454) -> (203.744, 226.3267)
  line L514 (226.7139, 193.2358) -> (225.9999, 194.0152)
  line L515 (222.5187, 198.0008) -> (221.8403, 198.8151)
  line L516 (199.9976, 233.9514) -> (199.1202, 235.8788)
  line L517 (182.5564, 293.5487) -> (182.2371, 295.7822)
  line L518 (180.4987, 311.6506) -> (180.4717, 311.679)
  line L519 (185.9971, 275.4966) -> (185.6552, 277.0009)
  line L520 (187.4627, 269.5009) -> (187.0815, 270.9964)
  line L521 (180.3952, 311.6873) -> (180.3057, 311.6671)
  line L522 (202.7719, 228.2187) -> (201.8234, 230.1206)
  line L523 (237.2155, 183.0945) -> (236.4487, 183.761)
  line L524 (227.4338, 192.4625) -> (226.7139, 193.2358)
  line L525 (190.8724, 257.6375) -> (190.4109, 259.1095)
  line L526 (183.8074, 286.0624) -> (183.533, 287.5775)
  line L527 (182.8997, 291.3191) -> (182.5564, 293.5487)
  line L528 (212.3736, 211.6361) -> (211.212, 213.4223)
  line L529 (219.1856, 202.126) -> (218.5367, 202.9667)
  line L530 (213.5589, 209.8663) -> (212.3736, 211.6361)
  line L531 (189.5182, 262.0636) -> (189.0871, 263.5453)
  line L532 (230.3726, 189.4324) -> (229.629, 190.1803)
  line L533 (189.0871, 263.5453) -> (188.666, 265.03)
  line L534 (214.7678, 208.1138) -> (213.5589, 209.8663)
  line L535 (244.3514, 177.3793) -> (243.5375, 177.987)
  line L536 (181.1766, 304.7448) -> (180.9601, 306.9902)
  line L537 (201.8234, 230.1206) -> (200.8986, 232.0318)
  line L538 (186.3487, 273.9944) -> (185.9971, 275.4966)
  line L539 (183.2681, 289.0936) -> (182.8997, 291.3191)
  line L540 (184.3848, 283.0359) -> (184.0913, 284.5485)
  line L541 (180.5721, 311.343) -> (180.5485, 311.4822)
  line L542 (180.3057, 311.6671) -> (180.2037, 311.6226)
  line L543 (185.3231, 278.5071) -> (185.0007, 280.0151)
  line L544 (241.9255, 179.2239) -> (241.1274, 179.8528)
  line L545 (185.0007, 280.0151) -> (184.6879, 281.5247)
  line L546 (185.6552, 277.0009) -> (185.3231, 278.5071)
  line L547 (188.507, 254.6357) -> (188.9622, 253.1172)
  line L548 (193.3337, 250.3316) -> (192.8209, 251.7851)
  line L549 (180.4351, 311.6869) -> (180.3952, 311.6873)
  line L550 (180.0897, 311.5578) -> (179.8267, 311.3836)
  line L551 (184.6879, 281.5247) -> (184.3848, 283.0359)
  line L552 (185.6118, 265.2959) -> (185.9946, 263.7713)
  line L553 (188.0623, 256.1558) -> (188.507, 254.6357)
  line L554 (181.2954, 286.3003) -> (181.6929, 283.9397)
  line L555 (178.6454, 310.3572) -> (178.6775, 309.7926)
  line L556 (183.4996, 274.5398) -> (184.0023, 272.2017)
  line L557 (183.0167, 276.8829) -> (183.4996, 274.5398)
  line L558 (180.2037, 311.6226) -> (180.0897, 311.5578)
  line L559 (181.9405, 298.019) -> (181.6657, 300.2587)
  line L560 (179.9406, 295.7767) -> (180.2427, 293.403)
  line L561 (194.3907, 247.4369) -> (193.857, 248.8821)
  line L562 (186.7907, 260.7229) -> (187.2042, 259.1996)
  line L563 (191.9162, 244.0497) -> (192.4462, 242.5478)
  line L564 (195.8561, 233.612) -> (196.4633, 232.1373)
  line L565 (199.6683, 224.8396) -> (200.3434, 223.3967)
  line L566 (178.6439, 310.5151) -> (178.6454, 310.3572)
  line L567 (181.6657, 300.2587) -> (181.4115, 302.5008)
  line L568 (203.1598, 217.6878) -> (203.893, 216.2773)
  line L569 (184.0913, 284.5485) -> (183.8074, 286.0624)
  line L570 (178.8531, 310.7789) -> (178.7652, 310.7155)
  line L571 (179.6638, 298.153) -> (179.9406, 295.7767)
  line L572 (178.6539, 310.5896) -> (178.6439, 310.5151)
  line L573 (180.7887, 308.9699) -> (180.6686, 310.4304)
  line L574 (180.6191, 310.957) -> (180.5721, 311.343)
  line L575 (178.9921, 305.295) -> (179.1889, 302.9124)
  line L576 (186.3875, 262.2469) -> (186.7907, 260.7229)
  line L577 (215.4145, 197.3775) -> (216.3292, 196.0967)
  line L578 (180.2427, 293.403) -> (180.5697, 291.0321)
  line L579 (189.9595, 260.5849) -> (189.5182, 262.0636)
  line L580 (184.8767, 268.345) -> (185.2392, 266.8206)
  line L581 (178.9593, 310.8452) -> (178.8531, 310.7789)
  line L582 (210.1861, 205.2683) -> (211.0269, 203.9297)
  line L583 (180.6686, 310.4304) -> (180.6191, 310.957)
  line L584 (192.3183, 253.2426) -> (191.8261, 254.7039)
  line L585 (187.0815, 270.9964) -> (186.7102, 272.4943)
  line L586 (178.8231, 307.6792) -> (178.9921, 305.295)
  line L587 (191.8261, 254.7039) -> (191.3441, 256.1689)
  line L588 (178.7652, 310.7155) -> (178.698, 310.653)
  line L589 (180.5697, 291.0321) -> (180.9207, 288.6645)
  line L590 (212.745, 201.2801) -> (213.6225, 199.9695)
  line L591 (206.944, 210.7088) -> (207.7365, 209.3361)
  line L592 (214.5123, 198.6685) -> (215.4145, 197.3775)
  line L593 (180.4717, 311.679) -> (180.4351, 311.6869)
  line L594 (186.7102, 272.4943) -> (186.3487, 273.9944)
  line L595 (179.2171, 310.994) -> (178.9593, 310.8452)
  line L596 (211.0269, 203.9297) -> (211.8798, 202.6003)
  line L597 (187.8539, 268.008) -> (187.4627, 269.5009)
  line L598 (192.8209, 251.7851) -> (192.3183, 253.2426)
  line L599 (181.4115, 302.5008) -> (181.1766, 304.7448)
  line L600 (180.5241, 311.5848) -> (180.4987, 311.6506)
  line L601 (178.698, 310.653) -> (178.6539, 310.5896)
  line L602 (188.2549, 266.5176) -> (187.8539, 268.008)
  line L603 (193.857, 248.8821) -> (193.3337, 250.3316)
  line L604 (182.2371, 295.7822) -> (181.9405, 298.019)
  line L605 (178.6775, 309.7926) -> (178.8231, 307.6792)
  line L606 (188.666, 265.03) -> (188.2549, 266.5176)
  line L607 (179.8267, 311.3836) -> (179.5198, 311.1773)
  line L608 (213.6225, 199.9695) -> (214.5123, 198.6685)
  line L609 (200.3434, 223.3967) -> (201.0301, 221.9599)
  line L610 (248.2795, 164.3452) -> (248.7417, 164.0152)
  line L611 (185.2392, 266.8206) -> (185.6118, 265.2959)
  line L612 (202.4383, 219.1052) -> (203.1598, 217.6878)
  line L613 (192.4462, 242.5478) -> (192.987, 241.0491)
  line L614 (182.1127, 281.5831) -> (182.5541, 279.2308)
  line L615 (190.8887, 247.0624) -> (191.3971, 245.5546)
  line L616 (222.0809, 188.6371) -> (223.0839, 187.4334)
  line L617 (258.1594, 184.4291) -> (259.3116, 185.3927)
  line L618 (216.3292, 196.0967) -> (217.2563, 194.8262)
  line L619 (218.196, 193.5664) -> (219.1482, 192.3173)
  line L620 (233.4201, 176.4745) -> (234.4601, 175.5038)
  line L621 (245.4149, 166.4368) -> (246.5604, 165.5962)
  line L622 (211.8798, 202.6003) -> (212.745, 201.2801)
  line L623 (206.1634, 212.0895) -> (206.944, 210.7088)
  line L624 (196.4633, 232.1373) -> (197.0816, 230.6674)
  line L625 (260.4544, 186.3677) -> (261.5885, 187.3529)
  line L626 (203.893, 216.2773) -> (204.638, 214.8739)
  line L627 (228.2925, 181.5975) -> (229.3732, 180.4683)
  line L628 (221.0906, 189.8524) -> (222.0809, 188.6371)
  line L629 (199.0045, 226.2884) -> (199.6683, 224.8396)
  line L630 (238.7259, 171.7356) -> (239.8176, 170.8226)
  line L631 (197.7113, 229.2025) -> (198.3522, 227.7427)
  line L632 (230.3674, 179.4533) -> (231.3735, 178.4493)
  line L633 (236.5723, 173.5967) -> (237.6441, 172.6603)
  line L634 (191.3971, 245.5546) -> (191.9162, 244.0497)
  line L635 (195.2602, 235.0912) -> (195.8561, 233.612)
  line L636 (224.0998, 186.2416) -> (225.1285, 185.0618)
  line L637 (179.4131, 300.5317) -> (179.6638, 298.153)
  line L638 (190.3911, 248.5727) -> (190.8887, 247.0624)
  line L639 (184.5243, 269.869) -> (184.8767, 268.345)
  line L640 (207.7365, 209.3361) -> (208.541, 207.9717)
  line L641 (194.6753, 236.5748) -> (195.2602, 235.0912)
  line L642 (197.0816, 230.6674) -> (197.7113, 229.2025)
  line L643 (187.2042, 259.1996) -> (187.6281, 257.6772)
  line L644 (208.541, 207.9717) -> (209.3575, 206.6157)
  line L645 (187.6281, 257.6772) -> (188.0623, 256.1558)
  line L646 (217.2563, 194.8262) -> (218.196, 193.5664)
  line L647 (252.5314, 180.0191) -> (253.5169, 180.7621)
  line L648 (256.997, 183.478) -> (258.1594, 184.4291)
  line L649 (267.467, 192.6714) -> (273.8913, 199.7292)
  line L650 (189.4279, 251.6003) -> (189.9042, 250.0855)
  line L651 (226.1702, 183.8944) -> (227.2248, 182.7396)
  line L652 (231.3735, 178.4493) -> (232.3911, 177.4563)
  line L653 (219.1482, 192.3173) -> (220.1131, 191.0792)
  line L654 (201.7284, 220.5293) -> (202.4383, 219.1052)
  line L655 (249.5354, 177.901) -> (249.6824, 177.9787)
  line L656 (198.3522, 227.7427) -> (199.0045, 226.2884)
  line L657 (188.9622, 253.1172) -> (189.4279, 251.6003)
  line L658 (189.9042, 250.0855) -> (190.3911, 248.5727)
  line L659 (193.5388, 239.5539) -> (194.1015, 238.0624)
  line L660 (201.0301, 221.9599) -> (201.7284, 220.5293)
  line L661 (180.9207, 288.6645) -> (181.2954, 286.3003)
  line L662 (204.638, 214.8739) -> (205.3948, 213.4779)
  line L663 (205.3948, 213.4779) -> (206.1634, 212.0895)
  line L664 (182.5541, 279.2308) -> (183.0167, 276.8829)
  line L665 (184.0023, 272.2017) -> (184.5243, 269.869)
  line L666 (194.1015, 238.0624) -> (194.6753, 236.5748)
  line L667 (185.9946, 263.7713) -> (186.3875, 262.2469)
  line L668 (209.3575, 206.6157) -> (210.1861, 205.2683)
  line L669 (250.973, 178.8699) -> (251.6831, 179.3885)
  line L670 (248.7417, 164.0152) -> (248.8743, 163.9263)
  line L671 (192.987, 241.0491) -> (193.5388, 239.5539)
  line L672 (181.6929, 283.9397) -> (182.1127, 281.5831)
  line L673 (255.8236, 182.5407) -> (256.997, 183.478)
  line L674 (290.6933, 223.8063) -> (296.4177, 234.9381)
  line L675 (282.6139, 211.0282) -> (283.5105, 212.3394)
  line L676 (244.2777, 167.2897) -> (245.4149, 166.4368)
  line L677 (312.5115, 285.2592) -> (312.8868, 287.2264)
  line L678 (262.7146, 188.3469) -> (263.8334, 189.3487)
  line L679 (249.9716, 178.1657) -> (250.4022, 178.4625)
  line L680 (300.6173, 244.7625) -> (301.4399, 246.861)
  line L681 (315.0267, 301.0632) -> (315.2623, 303.0467)
  line L682 (302.8475, 250.5937) -> (303.5267, 252.471)
  line L683 (243.1492, 168.1549) -> (244.2777, 167.2897)
  line L684 (266.5817, 191.8166) -> (267.0281, 192.2401)
  line L685 (274.9238, 200.9321) -> (275.9394, 202.1498)
  line L686 (259.3116, 185.3927) -> (260.4544, 186.3677)
  line L687 (261.5885, 187.3529) -> (262.7146, 188.3469)
  line L688 (232.3911, 177.4563) -> (233.4201, 176.4745)
  line L689 (246.5604, 165.5962) -> (248.2795, 164.3452)
  line L690 (220.1131, 191.0792) -> (221.0906, 189.8524)
  line L691 (309.8987, 273.5282) -> (310.3769, 275.4736)
  line L692 (225.1285, 185.0618) -> (226.1702, 183.8944)
  line L693 (309.4035, 271.5872) -> (309.8987, 273.5282)
  line L694 (316.2102, 312.8957) -> (316.2186, 313.1259)
  line L695 (223.0839, 187.4334) -> (224.0998, 186.2416)
  line L696 (308.8914, 269.6508) -> (309.4035, 271.5872)
  line L697 (284.3943, 213.6593) -> (285.2657, 214.9873)
  line L698 (304.8355, 256.246) -> (305.465, 258.1434)
  line L699 (265.6727, 190.9864) -> (266.5817, 191.8166)
  line L700 (235.5109, 174.5445) -> (236.5723, 173.5967)
  line L701 (251.6831, 179.3885) -> (252.5314, 180.0191)
  line L702 (275.9394, 202.1498) -> (276.9386, 203.3814)
  line L703 (303.5267, 252.471) -> (304.1894, 254.3551)
  line L704 (248.9417, 177.9125) -> (249.0871, 177.8762)
  line L705 (308.3623, 267.7194) -> (308.8914, 269.6508)
  line L706 (316.2158, 313.1958) -> (316.2081, 313.2354)
  line L707 (239.8176, 170.8226) -> (240.9189, 169.9214)
  line L708 (249.2381, 177.8615) -> (249.3893, 177.8694)
  line L709 (296.4177, 234.9381) -> (296.8337, 235.826)
  line L710 (254.6386, 181.6184) -> (255.8236, 182.5407)
  line L711 (315.2623, 303.0467) -> (315.4802, 305.0311)
  line L712 (248.8743, 163.9263) -> (248.9417, 163.8888)
  line L713 (276.9386, 203.3814) -> (277.9218, 204.6264)
  line L714 (249.3893, 177.8694) -> (249.5354, 177.901)
  line L715 (240.9189, 169.9214) -> (242.0295, 169.0321)
  line L716 (307.8164, 265.793) -> (308.3623, 267.7194)
  line L717 (297.8594, 238.1141) -> (298.4642, 239.516)
  line L718 (249.0871, 177.8762) -> (249.2381, 177.8615)
  line L719 (229.3732, 180.4683) -> (230.3674, 179.4533)
  line L720 (297.3151, 236.8844) -> (297.8594, 238.1141)
  line L721 (249.6824, 177.9787) -> (249.9716, 178.1657)
  line L722 (281.7039, 209.7265) -> (282.6139, 211.0282)
  line L723 (264.7525, 190.168) -> (265.6727, 190.9864)
  line L724 (253.5169, 180.7621) -> (254.6386, 181.6184)
  line L725 (316.2186, 313.1259) -> (316.2158, 313.1958)
  line L726 (306.6742, 261.9566) -> (307.2537, 263.872)
  line L727 (237.6441, 172.6603) -> (238.7259, 171.7356)
  line L728 (290.1953, 222.9368) -> (290.6933, 223.8063)
  line L729 (273.8913, 199.7292) -> (274.9238, 200.9321)
  line L730 (263.8334, 189.3487) -> (264.7525, 190.168)
  line L731 (267.0281, 192.2401) -> (267.467, 192.6714)
  line L732 (234.4601, 175.5038) -> (235.5109, 174.5445)
  line L733 (227.2248, 182.7396) -> (228.2925, 181.5975)
  line L734 (250.4022, 178.4625) -> (250.973, 178.8699)
  line L735 (242.0295, 169.0321) -> (243.1492, 168.1549)
  line L736 (291.2964, 325.8579) -> (289.4591, 326.4863)
  line L737 (296.7454, 323.8004) -> (295.8445, 324.1617)
  line L738 (314.5028, 297.1003) -> (314.7736, 299.081)
  line L739 (313.2448, 289.1964) -> (313.5854, 291.169)
  line L740 (315.8628, 309.0021) -> (316.0232, 310.7757)
  line L741 (316.0232, 310.7757) -> (316.1438, 312.0747)
  line L742 (311.2822, 279.3768) -> (311.7092, 281.3342)
  line L743 (275.9292, 330.2824) -> (275.5765, 330.3544)
  line L744 (262.5497, 332.3308) -> (261.5305, 332.4621)
  line L745 (301.199, 321.881) -> (300.3155, 322.2802)
  line L746 (312.087, 316.1005) -> (311.3889, 316.5222)
  line L747 (294.0336, 324.862) -> (293.1239, 325.2012)
  line L748 (316.2081, 313.2354) -> (316.1606, 313.3023)
  line L749 (314.2145, 295.1212) -> (314.5028, 297.1003)
  line L750 (304.6932, 320.206) -> (303.8259, 320.6366)
  line L751 (292.2114, 325.5331) -> (291.2964, 325.8579)
  line L752 (308.9614, 317.9317) -> (308.1173, 318.4029)
  line L753 (264.0974, 332.1374) -> (262.5497, 332.3308)
  line L754 (302.0787, 321.4741) -> (301.199, 321.881)
  line L755 (286.125, 216.3226) -> (286.9728, 217.6648)
  line L756 (315.4802, 305.0311) -> (315.6804, 307.0163)
  line L757 (310.3769, 275.4736) -> (310.8381, 277.4232)
  line L758 (293.1239, 325.2012) -> (292.2114, 325.5331)
  line L759 (276.462, 330.1653) -> (275.9292, 330.2824)
  line L760 (299.1271, 241.0907) -> (299.8456, 242.8393)
  line L761 (314.7736, 299.081) -> (315.0267, 301.0632)
  line L762 (316.1438, 312.0747) -> (316.2102, 312.8957)
  line L763 (278.8895, 205.884) -> (279.8422, 207.1537)
  line L764 (302.1519, 248.7237) -> (302.8475, 250.5937)
  line L765 (305.465, 258.1434) -> (306.0779, 260.047)
  line L766 (312.8868, 287.2264) -> (313.2448, 289.1964)
  line L767 (316.1606, 313.3023) -> (316.06, 313.4031)
  line L768 (313.5854, 291.169) -> (313.9087, 293.144)
  line L769 (288.6354, 220.3667) -> (289.6805, 222.0771)
  line L770 (283.5105, 212.3394) -> (284.3943, 213.6593)
  line L771 (313.9087, 293.144) -> (314.2145, 295.1212)
  line L772 (282.0331, 328.7248) -> (280.1625, 329.2181)
  line L773 (279.8422, 207.1537) -> (280.7801, 208.4347)
  line L774 (280.1625, 329.2181) -> (279.1067, 329.4948)
  line L775 (308.1173, 318.4029) -> (307.2683, 318.8659)
  line L776 (259.4904, 332.7106) -> (258.979, 332.7568)
  line L777 (294.9406, 324.5155) -> (294.0336, 324.862)
  line L778 (316.06, 313.4031) -> (315.906, 313.5369)
  line L779 (299.4283, 322.6717) -> (298.5374, 323.0555)
  line L780 (315.6804, 307.0163) -> (315.8628, 309.0021)
  line L781 (275.5765, 330.3544) -> (274.849, 330.4954)
  line L782 (307.2537, 263.872) -> (307.8164, 265.793)
  line L783 (277.9218, 204.6264) -> (278.8895, 205.884)
  line L784 (299.8456, 242.8393) -> (300.6173, 244.7625)
  line L785 (311.7092, 281.3342) -> (312.1189, 283.295)
  line L786 (304.1894, 254.3551) -> (304.8355, 256.246)
  line L787 (287.8094, 219.013) -> (288.6354, 220.3667)
  line L788 (286.9728, 217.6648) -> (287.8094, 219.013)
  line L789 (301.4399, 246.861) -> (302.1519, 248.7237)
  line L790 (306.0779, 260.047) -> (306.6742, 261.9566)
  line L791 (285.2657, 214.9873) -> (286.125, 216.3226)
  line L792 (312.1189, 283.295) -> (312.5115, 285.2592)
  line L793 (289.6805, 222.0771) -> (290.1953, 222.9368)
  line L794 (310.8381, 277.4232) -> (311.2822, 279.3768)
  line L795 (280.7801, 208.4347) -> (281.7039, 209.7265)
  line L796 (298.4642, 239.516) -> (299.1271, 241.0907)
  line L797 (296.8337, 235.826) -> (297.3151, 236.8844)
  line L798 (311.3889, 316.5222) -> (310.6354, 316.9685)
  line L799 (232.3697, 331.8744) -> (231.3075, 331.7228)
  line L800 (182.399, 313.3626) -> (182.3741, 313.2667)
  line L801 (230.2571, 331.5647) -> (229.2183, 331.4005)
  line L802 (182.3576, 312.5288) -> (182.3964, 311.6644)
  line L803 (265.5496, 331.948) -> (264.0974, 332.1374)
  line L804 (261.5305, 332.4621) -> (260.5112, 332.5947)
  line L805 (309.8263, 317.4386) -> (308.9614, 317.9317)
  line L806 (237.1655, 332.5067) -> (234.9862, 332.2301)
  line L807 (315.906, 313.5369) -> (315.6984, 313.7029)
  line L808 (283.8991, 328.2054) -> (282.0331, 328.7248)
  line L809 (303.8259, 320.6366) -> (302.9543, 321.0593)
  line L810 (307.2683, 318.8659) -> (306.4145, 319.3207)
  line L811 (272.2648, 330.9515) -> (270.406, 331.2502)
  line L812 (310.6354, 316.9685) -> (309.8263, 317.4386)
  line L813 (258.4667, 332.792) -> (240.2104, 332.8044)
  line L814 (273.7454, 330.6972) -> (272.2648, 330.9515)
  line L815 (314.3287, 314.6744) -> (313.3176, 315.3337)
  line L816 (260.5112, 332.5947) -> (259.4904, 332.7106)
  line L817 (234.9862, 332.2301) -> (232.3697, 331.8744)
  line L818 (315.4371, 313.9005) -> (315.1218, 314.1288)
  line L819 (227.1757, 331.054) -> (226.1718, 330.8721)
  line L820 (313.3176, 315.3337) -> (312.087, 316.1005)
  line L821 (306.4145, 319.3207) -> (305.5561, 319.7674)
  line L822 (287.6132, 327.0866) -> (285.7595, 327.6595)
  line L823 (279.1067, 329.4948) -> (278.0512, 329.7733)
  line L824 (182.7661, 307.3054) -> (182.9779, 305.2707)
  line L825 (182.9779, 305.2707) -> (183.2362, 302.9484)
  line L826 (285.7595, 327.6595) -> (283.8991, 328.2054)
  line L827 (305.5561, 319.7674) -> (304.6932, 320.206)
  line L828 (224.199, 330.492) -> (222.2726, 330.0911)
  line L829 (270.406, 331.2502) -> (268.1679, 331.5851)
  line L830 (258.979, 332.7568) -> (258.4667, 332.792)
  line L831 (298.5374, 323.0555) -> (297.6431, 323.4317)
  line L832 (240.2104, 332.8044) -> (239.6136, 332.7633)
  line L833 (302.9543, 321.0593) -> (302.0787, 321.4741)
  line L834 (238.9071, 332.6996) -> (238.0911, 332.6139)
  line L835 (238.0911, 332.6139) -> (237.1655, 332.5067)
  line L836 (274.849, 330.4954) -> (273.7454, 330.6972)
  line L837 (297.6431, 323.4317) -> (296.7454, 323.8004)
  line L838 (216.77, 328.7785) -> (215.0276, 328.3091)
  line L839 (189.5942, 317.9397) -> (188.7829, 317.4811)
  line L840 (222.2726, 330.0911) -> (220.3923, 329.671)
  line L841 (289.4591, 326.4863) -> (287.6132, 327.0866)
  line L842 (315.1218, 314.1288) -> (314.3287, 314.6744)
  line L843 (239.6136, 332.7633) -> (238.9071, 332.6996)
  line L844 (206.9983, 325.7856) -> (205.528, 325.2557)
  line L845 (218.5582, 329.233) -> (216.77, 328.7785)
  line L846 (188.7829, 317.4811) -> (187.2886, 316.6135)
  line L847 (315.6984, 313.7029) -> (315.4371, 313.9005)
  line L848 (295.8445, 324.1617) -> (294.9406, 324.5155)
  line L849 (182.4765, 310.5043) -> (182.5993, 309.0506)
  line L850 (220.3923, 329.671) -> (218.5582, 329.233)
  line L851 (200.0942, 323.0985) -> (198.8469, 322.5569)
  line L852 (278.0512, 329.7733) -> (276.9931, 330.0404)
  line L853 (300.3155, 322.2802) -> (299.4283, 322.6717)
  line L854 (197.6438, 322.0173) -> (196.4848, 321.481)
  line L855 (268.1679, 331.5851) -> (265.5496, 331.948)
  line L856 (182.3741, 313.2667) -> (182.3588, 313.0956)
  line L857 (208.5136, 326.3091) -> (206.9983, 325.7856)
  line L858 (183.7282, 298.9665) -> (184.0014, 296.9774)
  line L859 (201.3858, 323.6405) -> (200.0942, 323.0985)
  line L860 (183.4731, 300.9569) -> (183.7282, 298.9665)
  line L861 (184.0014, 296.9774) -> (184.2925, 294.9899)
  line L862 (276.9931, 330.0404) -> (276.462, 330.1653)
  line L863 (215.0276, 328.3091) -> (213.3309, 327.826)
  line L864 (217.9652, 208.1433) -> (218.8395, 206.9696)
  line L865 (226.269, 197.912) -> (227.251, 196.8254)
  line L866 (234.4449, 189.5439) -> (235.5173, 188.5534)
  line L867 (193.1466, 257.8179) -> (193.7823, 255.9081)
  line L868 (197.2058, 246.4567) -> (197.9391, 244.5874)
  line L869 (184.5455, 314.8912) -> (183.6557, 314.2798)
  line L870 (202.7219, 324.1817) -> (201.3858, 323.6405)
  line L871 (185.2733, 289.0389) -> (185.6357, 287.0598)
  line L872 (184.6016, 293.0042) -> (184.9285, 291.0204)
  line L873 (187.7108, 277.2089) -> (188.178, 275.2492)
  line L874 (242.1796, 182.8983) -> (243.1905, 182.1136)
  line L875 (196.4848, 321.481) -> (195.3697, 320.9495)
  line L876 (186.3635, 316.0568) -> (185.4486, 315.4831)
  line L877 (182.5993, 309.0506) -> (182.7661, 307.3054)
  line L878 (183.6557, 314.2798) -> (182.734, 313.6258)
  line L879 (193.2708, 319.9065) -> (192.2867, 319.3977)